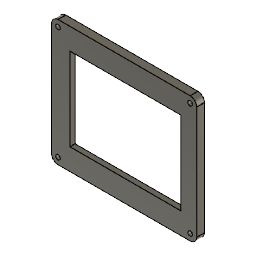
Front-Display-0 (Autodesk Fusion 360 design; units mm, degrees)
part number: 2026-02-02-21-42-42-958
Autodesk Fusion 360 part; units mm, degrees
sketch "Sketch1" plane through (0, 0, 0) normal (0, 1, 0) x (1, 0, 0)
  line L0 (908.9213, 286.0768) -> (797.9213, 286.0768)
  line L1 (797.9213, 286.0768) -> (797.9213, 382.2768)
  line L2 (797.9213, 382.2768) -> (908.9213, 382.2768)
  line L3 (908.9213, 382.2768) -> (908.9213, 286.0768)
  line L4 (894.8127, 302.485) -> (810.0127, 302.485)
  line L5 (810.0127, 302.485) -> (810.0127, 365.785)
  line L6 (810.0127, 365.785) -> (894.8127, 365.785)
  line L7 (894.8127, 365.785) -> (894.8127, 302.485)
  circle A0 centre (903.9213, 377.2768) radius 1.75
  circle A1 centre (802.9213, 377.2768) radius 1.75
  circle A2 centre (802.9213, 291.0768) radius 1.75
  circle A3 centre (903.9213, 291.0768) radius 1.75
  dimension "d1" = 96.2
  dimension "d2" = 111
  dimension "d7" = 84.8
  dimension "d8" = 63.3
  dimension "d9" = 5
  dimension "d10" = 5
  dimension "d11" = 3.5
  dimension "d12" = 3.5
  dimension "d13" = 5
  dimension "d14" = 5
  dimension "d15" = 3.5
  dimension "d16" = 5
  dimension "d17" = 5
  dimension "d18" = 3.5
  dimension "d19" = 5
  dimension "d20" = 5
  constraint horizontal L0
  constraint vertical L1
  constraint horizontal L2
  constraint vertical L3
  constraint horizontal L4
  constraint vertical L5
  constraint horizontal L6
  constraint vertical L7
  measures "d1" distance of L0 L2
  measures "d2" distance of L1 L3
  measures "d7" distance of L5 L7
  measures "d8" distance of L4 L6
  measures "d9" distance of L2 A0.centre
  measures "d10" distance of L3 A0.centre
  measures "d11" diameter of A0
  measures "d12" diameter of A1
  measures "d13" distance of L1 A1.centre
  measures "d14" distance of L2 A1.centre
  measures "d15" diameter of A2
  measures "d16" distance of L1 A2.centre
  measures "d17" distance of L0 A2.centre
  measures "d18" diameter of A3
  measures "d19" distance of L0 A3.centre
  measures "d20" distance of L3 A3.centre
extrude "Extrude1" add sketch "Sketch1" along normal blind 6
sketch "Sketch2" plane through (0, 0, 0) normal (0, -1, 0) x (1, 0, 0)
  circle A0 centre (903.9213, -377.2768) radius 1.75
  circle A1 centre (802.9213, -377.2768) radius 1.75
  line L0 (894.8127, -365.785) -> (810.0127, -365.785)
  line L1 (810.0127, -365.785) -> (810.0127, -302.485)
  line L2 (810.0127, -302.485) -> (894.8127, -302.485)
  line L3 (894.8127, -302.485) -> (894.8127, -365.785)
  circle A2 centre (802.9213, -291.0768) radius 1.75
  circle A3 centre (903.9213, -291.0768) radius 1.75
  line L4 (797.9213, -382.2768) -> (908.9213, -382.2768)
  line L5 (908.9213, -382.2768) -> (908.9213, -286.0768)
  line L6 (908.9213, -286.0768) -> (797.9213, -286.0768)
  line L7 (797.9213, -286.0768) -> (797.9213, -382.2768)
  line L8 (806.6966, -298.2951) -> (898.0588, -298.2951)
  line L9 (898.0588, -298.2951) -> (898.0588, -377.458)
  line L10 (898.0588, -377.458) -> (806.6966, -377.458)
  line L11 (806.6966, -377.458) -> (806.6966, -298.2951)
  dimension "d23" = 79.1629
  dimension "d24" = 91.3622
  constraint horizontal L8
  constraint vertical L9
  constraint horizontal L10
  constraint vertical L11
  measures "d23" distance of L8 L10
  measures "d24" distance of L9 L11
extrude "Extrude2" cut sketch "Sketch2" against normal blind 2 contours L8 L9 L10 L11
move_body "Move1" bodies 1 to x (1, 0, 0) y (0, 1, 0) z (0, 0, 1) at (-546.9712, 0, 227.1574)
move_body "Move2" bodies 1 to x (1, 0, 0) y (0, 1, 0) z (0, 0, 1) at (-128.0537, 0, 130.0546)
move_body "Move3" bodies 1 to x (-1, 0, 0) y (0, -1, 0) z (0, 0, 1) at (171.4369, 2, -21.0966)
fillet "Fillet1" radius 5 1 edges at (48.5405, -1, 50.0386)
fillet "Fillet2" radius 5 1 edges at (48.5405, -1, -46.1614)
fillet "Fillet3" radius 5 1 edges at (-62.4595, -1, -46.1614)
fillet "Fillet4" radius 5 1 edges at (-62.4595, -1, 50.0386)
